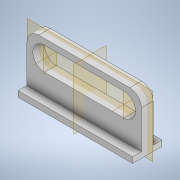
# Autodesk Inventor part: PistaEslabonPreliminar
Saved by Autodesk Inventor 2021 (Build 250183000, 183)
## iProperties
Created: 2021-04-17
Part Number: PistaEslabonPreliminar
Material: Generic
Document SubType Name: Modeling
Designer: GABRIEL LOL
Density: 1 g/cm^3
Appearance: Default
Mass: 36.7642 g
Surface Area: 137.908 cm^2
Volume: 36.7642 cm^3
Author: GABRIEL LOL
Autodesk Inventor part; units mm, degrees
ref_plane "YZ Plane" through (0, 0, 0) normal (1, 0, 0) x (0, 1, 0)
ref_plane "XZ Plane" through (0, 0, 0) normal (0, 1, 0) x (-1, 0, 0)
ref_plane "XY Plane" through (0, 0, 0) normal (0, 0, 1) x (1, 0, 0)
sketch "Sketch1" plane through (0, 0, 0) normal (0, 0, 1) x (1, 0, 0)
  line L0 (0, 0) -> (68.1, 0)
  circle A0 centre (0, 0) radius 10
  circle A1 centre (68.1, 0) radius 10
  line L1 (0, 10) -> (68.1, 10)
  line L2 (0, -10) -> (68.1, -10)
  circle A2 centre (0, 0) radius 15
  circle A3 centre (68.1, 0) radius 15
  line L3 (0, 15) -> (68.1, 15)
  line L4 (68.1, -15) -> (0, -15)
  dimension "d0" = 68.1
  dimension "d1" = 20
  dimension "d2" = 20
  dimension "d3" = 30
  dimension "d4" = 30
  constraints: 10 end point, 8 point on circle, 5 tangent, 4 centre point, 4 coincident, 1 horizontal
  measures "d0" distance of L0.start L0.end
  measures "d1" diameter of A0
  measures "d2" diameter of A1
  measures "d3" diameter of A2
  measures "d4" diameter of A3
extrude "Extrusion1" add sketch "Sketch1" along normal blind 10 contours A0 L2 A2 L1 | A2 L3 A3 L1 | L2 A3 L4 A2 | A3 L2 A1 L1
sketch "Sketch2" plane through (0, 0, 10) normal (0, 0, 1) x (1, 0, 0)
  line L0 (0, 0) -> (0, -32.5) construction
  arc A0 (0, 15) -> (0, -15) centre (0, 0) ccw construction
  line L1 (-15, 0) -> (-15, -32.5) construction
  arc A1 (68.1, -15) -> (68.1, 15) centre (68.1, 0) ccw construction
  line L2 (83.1, 0) -> (83.1, -32.5) construction
  line L3 (-15, -32.5) -> (-15, 15)
  line L4 (-15, 15) -> (83.1, 15)
  line L5 (83.1, 15) -> (83.1, -32.5)
  line L6 (83.1, -32.5) -> (-15, -32.5)
  line L7 (0, 10) -> (68.1, 10) projected
  arc A2 (0, 10) -> (0, -10) centre (0, 0) ccw projected
  line L8 (68.1, -10) -> (0, -10) projected
  arc A3 (68.1, -10) -> (68.1, 10) centre (68.1, 0) ccw projected
  dimension "d7" = 32.5
  constraints: 14 end point, 3 vertical, 2 parallel, 2 point on circle, 2 tangent, 1 perpendicular, 1 point on line
  measures "d7" distance of L0.start L0.end
extrude "Extrusion2" add sketch "Sketch2" against normal blind 10
fillet "Fillet1" radius 10 1 edges at (83.1, 15, 5)
fillet "Fillet2" radius 10 1 edges at (-15, 15, 5)
ref_plane "Work Plane1" through (0, 0, 5) normal (0, 0, 1) x (1, 0, 0)
sketch "Sketch3" plane through (0, 0, 5) normal (0, 0, 1) x (1, 0, 0)
  arc A0 (-5, 15) -> (-15, 5) centre (-5, 5) ccw projected
  line L0 (-5, 15) -> (73.1, 15) projected
  line L1 (83.1, 5) -> (83.1, -32.5) projected
  line L2 (83.1, -32.5) -> (-15, -32.5) projected
  line L3 (-15, -32.5) -> (-15, 5) projected
  line L4 (0, 10) -> (68.1, 10) projected
  arc A1 (0, 10) -> (0, -10) centre (0, 0) ccw projected
  line L5 (68.1, -10) -> (0, -10) projected
  arc A2 (68.1, -10) -> (68.1, 10) centre (68.1, 0) ccw projected
  line L6 (83.1, -32.5) -> (-15, -32.5) projected
  line L7 (-15, -32.5) -> (83.1, -32.5)
  line L8 (83.1, -32.5) -> (83.1, -27.5)
  line L9 (83.1, -27.5) -> (-15, -27.5)
  line L10 (-15, -27.5) -> (-15, -32.5)
  arc A3 (83.1, 5) -> (73.1, 15) centre (73.1, 5) ccw projected
  dimension "d12" = 5
  constraints: 8 end point, 3 equal length, 1 perpendicular
  measures "d12" distance of L8.end L6.start
extrude "Extrusion3" add sketch "Sketch3" along normal mid plane 25 contours L9 L1 L2 L3
ref_plane "Work Plane2" through (68.1, -10, 10) normal (1, 0, 0) x (0, 0, -1)
ref_plane "Work Plane3" through (0, -10, 10) normal (1, 0, 0) x (0, 0, -1)
ref_plane "Work Plane4" through (34.05, 5, 10) normal (1, 0, 0) x (0, 0, -1)
body "Solid1"
